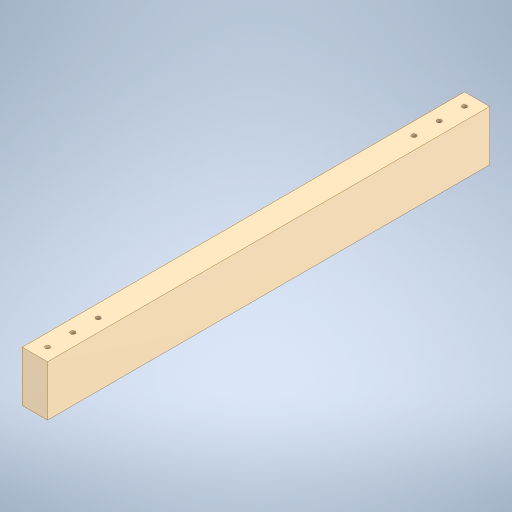
# Autodesk Inventor part: Chassis Bar
Saved by Autodesk Inventor 2023.4 (Build 274418000, 418)
## iProperties
Created: 2023-12-26
Part Number: Chassis Bar
Material: Polyethylene, High Density
Document SubType Name: Modeling
Designer: amrom
Density: 0.952 g/cm^3
Appearance: Smooth - Off-White
Mass: 619.413 g
Surface Area: 841.143 cm^2
Volume: 650.644 cm^3
Author: amrom
Autodesk Inventor part; units mm, degrees
ref_plane "YZ Plane" through (0, 0, 0) normal (1, 0, 0) x (0, 1, 0)
ref_plane "XZ Plane" through (0, 0, 0) normal (0, 1, 0) x (-1, 0, 0)
ref_plane "XY Plane" through (0, 0, 0) normal (0, 0, 1) x (1, 0, 0)
sketch "Sketch2" plane through (0, 0, 0) normal (0, 0, 1) x (1, 0, 0)
  line L0 (0, 0) -> (25.4, 0)
  line L1 (25.4, 0) -> (25.4, -50.8)
  line L2 (25.4, -50.8) -> (0, -50.8)
  line L3 (0, -50.8) -> (0, 0)
  dimension "d4" = 25.4
  dimension "d5" = 50.8
  constraints: 8 end point, 2 parallel, 1 horizontal, 1 perpendicular
  measures "d4" distance of L1.end L2.end
  measures "d5" distance of L0.end L1.end
extrude "Extrusion2" add sketch "Sketch2" along normal blind 444.5
sketch "Sketch3" plane through (0, 0, 0) normal (0, 1, 0) x (1, 0, 0)
  circle A0 centre (12.7, -431.8) radius 2.2479
  line L0 (0, 0) -> (0, -444.5) projected
  line L1 (25.4, -444.5) -> (0, -444.5) projected
  circle A1 centre (12.7, -406.4) radius 2.2479
  circle A2 centre (12.7, -381) radius 2.2479
  dimension "d8" = 4.4958
  dimension "d9" = 12.7
  dimension "d10" = 12.7
  dimension "d13" = 25.4
  constraints: 3 centre point, 1 vertical, 4 other
  measures "d8" diameter of A0
  measures "d9" distance from line of L0 A0.centre
  measures "d10" distance from line of L1 A0.centre
  measures "d13" distance of A0.centre A1.centre
extrude "Extrusion3" cut sketch "Sketch3" against normal blind 609.6
sketch "Sketch4" plane through (0, 0, 0) normal (0, 1, 0) x (1, 0, 0)
  circle A0 centre (12.7, -12.7) radius 2.2479
  line L0 (25.4, 0) -> (0, 0) projected
  line L1 (25.4, 0) -> (25.4, -444.5) projected
  circle A1 centre (12.7, -38.1) radius 2.2479
  circle A2 centre (12.7, -63.5) radius 2.2479
  dimension "d20" = 4.4958
  dimension "d21" = 12.7
  dimension "d22" = 12.7
  dimension "d25" = 25.4
  constraints: 3 centre point, 1 vertical, 4 other
  measures "d20" diameter of A0
  measures "d21" distance from line of L0 A0.centre
  measures "d22" distance from line of L1 A0.centre
  measures "d25" distance of A0.centre A1.centre
extrude "Extrusion4" cut sketch "Sketch4" against normal blind 609.6
body "Solid2"
